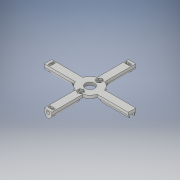
# Autodesk Inventor part: BrImp_Bridge
Saved by Autodesk Inventor 2018 (Build 220112000, 112)
## iProperties
Created: 2018-02-04
Part Number: BrImp_Bridge
Material: Generic
Document SubType Name: Modeling
Designer: Benedikt
Density: 1 g/cm^3
Appearance: Default
Author: Benedikt
Autodesk Inventor part; units mm, degrees
note: some values were not read from the file. Chosen so that the rebuilt part matches the saved one: direction of "Hole1".
ref_plane "YZ Plane" through (0, 0, 0) normal (1, 0, 0) x (0, 1, 0)
ref_plane "XZ Plane" through (0, 0, 0) normal (0, 1, 0) x (-1, 0, 0)
ref_plane "XY Plane" through (0, 0, 0) normal (0, 0, 1) x (1, 0, 0)
sketch "Sketch1" plane through (0, 0, 0) normal (0, 0, 1) x (1, 0, 0)
  circle A0 centre (0, 0) radius 4.1 projected
  arc A1 (4.1, -11.8085) -> (11.8085, -4.1) centre (0, 0) ccw projected
  circle A2 centre (0, 0) radius 12.3
  circle A3 centre (0, 0) radius 5
  point P0 (0, 0)
  dimension "d0" = 24.6
  dimension "d1" = 10
  constraints: 2 centre point, 2 coincident
  measures "d0" diameter of A2
  measures "d1" diameter of A3
extrude "Extrusion1" add sketch "Sketch1" along normal blind 3 contours A2
sketch "Sketch2" plane through (0, 0, 0) normal (0, 0, -1) x (-1, 0, 0)
  circle A0 centre (0, 0) radius 12.3 projected
  line L0 (4, -45) -> (-4, -45)
  line L1 (-4, 45) -> (4, 45)
  circle A1 centre (0, 0) radius 5 projected
  line L2 (-4, -45) -> (-4, -11.6314)
  line L3 (-4, 11.6314) -> (-4, 45)
  line L4 (4, -45) -> (0.4427, -4.9804) construction
  line L5 (-0.4427, 4.9804) -> (-4, 45) construction
  line L6 (-4, -45) -> (-0.4427, -4.9804) construction
  line L7 (0.4427, 4.9804) -> (4, 45) construction
  line L8 (4, -11.6314) -> (4, -45)
  line L9 (45, -4) -> (45, 4)
  line L10 (-45, 4) -> (-45, -4)
  line L11 (-45, -4) -> (45, 4) construction
  line L12 (45, -4) -> (-45, 4) construction
  line L13 (-11.6314, 4) -> (-45, 4)
  line L14 (4, 45) -> (4, 11.6314)
  line L15 (45, 4) -> (11.6314, 4)
  line L16 (11.6314, -4) -> (45, -4)
  line L17 (-45, -4) -> (-11.6314, -4)
  point P0 (0, 0)
  dimension "d4" = 8
  dimension "d5" = 90
  dimension "d6" = 90
  dimension "d7" = 8
  constraints: 36 end point, 10 parallel, 4 perpendicular, 4 point on circle, 3 horizontal, 2 midpoint, 9 other
  measures "d4" distance of L1.start L1.end
  measures "d5" distance of L0.end L1.start
  measures "d6" distance of L10.start L9.end
  measures "d7" distance of L9.end L9.start
extrude "Extrusion2" add sketch "Sketch2" against normal blind 3 contours A0 L15 L9 L16 | A0 L3 L1 L14 | L8 L0 L2 A0 | A0 L17 L10 L13
sketch "Sketch3" plane through (0, 0, 3) normal (0, 0, 1) x (1, 0, 0)
  circle A0 centre (0, -10) radius 1.7 projected
  circle A1 centre (0, 10) radius 1.7 projected
  line L0 (0, -6.6514) -> (2.9, -8.3257)
  line L1 (2.9, -8.3257) -> (2.9, -11.6743)
  line L2 (2.9, -11.6743) -> (0, -13.3486)
  line L3 (0, -13.3486) -> (-2.9, -11.6743)
  line L4 (-2.9, -11.6743) -> (-2.9, -8.3257)
  line L5 (-2.9, -8.3257) -> (0, -6.6514)
  line L6 (0, 13.3486) -> (2.9, 11.6743)
  line L7 (2.9, 11.6743) -> (2.9, 8.3257)
  line L8 (2.9, 8.3257) -> (0, 6.6514)
  line L9 (0, 6.6514) -> (-2.9, 8.3257)
  line L10 (-2.9, 8.3257) -> (-2.9, 11.6743)
  line L11 (-2.9, 11.6743) -> (0, 13.3486)
  point P0 (0, 0)
  dimension "d10" = 5.8
  dimension "d11" = 5.8
  constraints: 24 end point, 2 coincident, 26 other
  measures "d10" distance between parallel lines of L1 L4
  measures "d11" distance between parallel lines of L7 L10
extrude "Extrusion3" cut sketch "Sketch3" against normal blind 2 contours A0 | A1 | L0 L1 L2 L3 L4 L5 | L6 L7 L8 L9 L10 L11
sketch "Sketch4" plane through (0, 0, 1) normal (0, 0, 1) x (1, 0, 0)
  line L0 (0, 13.3486) -> (2.9, 11.6743) projected
  line L1 (-2.9, 11.6743) -> (0, 13.3486) projected
  line L2 (-2.9, 8.3257) -> (-2.9, 11.6743) projected
  line L3 (0, 6.6514) -> (-2.9, 8.3257) projected
  line L4 (2.9, 8.3257) -> (0, 6.6514) projected
  line L5 (2.9, 11.6743) -> (2.9, 8.3257) projected
  line L6 (0, -6.6514) -> (2.9, -8.3257) projected
  line L7 (-2.9, -8.3257) -> (0, -6.6514) projected
  line L8 (-2.9, -11.6743) -> (-2.9, -8.3257) projected
  line L9 (0, -13.3486) -> (-2.9, -11.6743) projected
  line L10 (2.9, -11.6743) -> (0, -13.3486) projected
  line L11 (2.9, -8.3257) -> (2.9, -11.6743) projected
  point P0 (0, 0)
  point P1 (0, 10)
  point P2 (0, -10)
hole "Hole1" at (0, 10, 1) at (0, -10, 1) direction (0, 0, -1) diameter 3.4 end up to surface
sketch "Sketch5" plane through (0, 0, 0) normal (0, 0, -1) x (-1, 0, 0)
  line L0 (-4, -14.975) -> (-4, -45)
  line L1 (4, -45) -> (4, -14.975)
  line L2 (11.6314, -4) -> (45, -4) projected
  line L3 (45, -4) -> (45, 4) projected
  line L4 (45, 4) -> (11.6314, 4) projected
  line L5 (4, 11.6314) -> (4, 45) projected
  line L6 (4, 45) -> (-4, 45) projected
  line L7 (-4, 45) -> (-4, 11.6314) projected
  line L8 (-11.6314, 4) -> (-45, 4) projected
  line L9 (-45, 4) -> (-45, -4) projected
  line L10 (-45, -4) -> (-11.6314, -4) projected
  circle A0 centre (0, 0) radius 15.5
  line L11 (-4, -45) -> (4, -45)
  point P0 (0, 0)
  dimension "d21" = 31
  constraints: 6 end point, 2 point on circle, 1 centre point, 1 horizontal
  measures "d21" diameter of A0
extrude "Extrusion4" add sketch "Sketch5" along normal blind 4.75 contours A0 L1 L11 L0
sketch "Sketch7" plane through (-4, -45, 3) normal (0, -1, 0) x (1, 0, 0)
  line L0 (4, -7.7009) -> (6.8804, -7.0425) construction
  line L1 (8, 0) -> (8, -7.75) projected
  line L2 (6.8804, -7.0425) -> (8, -3) construction
  spline S0 degree 2 poles (4, -7.7009) (6.8804, -7.0425) (8, -3) knots 1 1 1 2 2 2
  line L3 (4, -3) -> (4, -11.3047) construction
  line L4 (4, -7.7009) -> (1.1196, -7.0425) construction
  line L5 (1.1196, -7.0425) -> (0, -3) construction
  spline S1 degree 2 poles (4, -7.7009) (1.1196, -7.0425) (0, -3) knots 1 1 1 2 2 2
  line L6 (8, -3) -> (8, -7.75)
  line L7 (0, -7.75) -> (0, 0) projected
  line L8 (0, -7.75) -> (0, -3)
  line L9 (8, -7.75) -> (0, -7.75) projected
  line L10 (8, -7.75) -> (0, -7.75)
  constraints: 8 end point, 2 collinear, 2 symmetric about line, 1 horizontal, 1 point on line, 1 vertical, 6 other
extrude "Extrusion5" cut sketch "Sketch7" against normal blind 31.75
pattern_circular "Circular Pattern2" count 4 over 360 about axis through (0, 0, 0) along (0, 0, 1) of "Extrusion4", "Extrusion5"
sketch "Sketch8" plane through (45, -4, 3) normal (1, 0, 0) x (0, 0, -1)
  line L0 (3.2115, 6.4449) -> (9.2115, 6.4449)
  line L1 (9.2115, 6.4449) -> (9.2115, 1.4449)
  line L2 (9.2115, 1.4449) -> (3.2115, 1.4449)
  line L3 (3.2115, 1.4449) -> (3.2115, 6.4449)
  line L4 (3.2115, 6.4449) -> (9.2115, 1.4449) construction
  line L5 (9.2115, 6.4449) -> (3.2115, 1.4449) construction
  point P0 (3, 4)
  point P1 (6.2115, 3.9449)
  dimension "d34" = 6
  dimension "d35" = 5
  constraints: 12 end point, 2 midpoint, 2 parallel, 1 horizontal, 1 perpendicular
  measures "d34" distance between parallel lines of L3 L1
  measures "d35" distance of L2.end L0.start
extrude "Extrusion6" cut sketch "Sketch8" against normal blind 31.75
sketch "Sketch11" plane through (-4, -45, 3) normal (0, -1, 0) x (1, 0, 0)
  circle A0 centre (4, -2.5) radius 1.7
  line L0 (0, 0) -> (8, 0) projected
  point P0 (4, -3)
  dimension "d39" = 3.4
  dimension "d40" = 2.5
  constraints: 1 centre point
  measures "d39" diameter of A0
  measures "d40" distance from line of L0 A0.centre
extrude "Extrusion8" cut sketch "Sketch11" against normal blind 25
sketch "Sketch12" plane through (0, 0, 3) normal (0, 0, 1) x (1, 0, 0)
  line L0 (2.9, -42.3736) -> (-2.9, -42.3736)
  line L1 (-2.9, -42.3736) -> (-2.9, -39.6736)
  line L2 (-2.9, -39.6736) -> (2.9, -39.6736)
  line L3 (2.9, -39.6736) -> (2.9, -42.3736)
  line L4 (0, -45) -> (0, -15.5) projected
  line L5 (2.9, -42.3736) -> (-2.9, -39.6736) construction
  line L6 (-2.9, -42.3736) -> (2.9, -39.6736) construction
  point P0 (0, 0)
  point P1 (0, -41.0236)
  dimension "d43" = 5.8
  dimension "d44" = 2.7
  constraints: 12 end point, 2 midpoint, 2 parallel, 1 horizontal, 1 perpendicular, 1 point on line
  measures "d43" distance of L1.end L2.end
  measures "d44" distance of L0.end L1.end
extrude "Extrusion9" cut sketch "Sketch12" against normal blind 8.2
sketch "Sketch9" plane through (0, 0, 3) normal (0, 0, 1) x (1, 0, 0)
  line L0 (-45, 0) -> (-15.5, 0) projected
  circle A0 centre (0, 0) radius 45
  circle A1 centre (0, 0) radius 70.0494
  constraints: 2 coincident, 1 centre point, 1 horizontal alignment, 2 other
extrude "Extrusion7" cut sketch "Sketch9" against normal blind 31.75
pattern_circular "Circular Pattern3" count 3 over 180 about axis through (0, 0, 0) along (0, 0, -1) of "Extrusion8", "Extrusion9"
body "Solid1"
